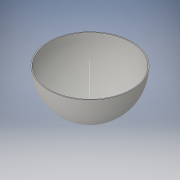
# Autodesk Inventor part: roundSaladBowl
Saved by Autodesk Inventor 2016 SP1 (Build 200210100, 210)
## iProperties
Created: 2016-01-19
Part Number: roundSaladBowl
Material: Generic
Document SubType Name: Modeling
Designer: steele
Density: 1 g/cm^3
Appearance: Default
Author: steele
Autodesk Inventor part; units mm, degrees
ref_plane "YZ Plane" through (0, 0, 0) normal (1, 0, 0) x (0, 1, 0)
ref_plane "XZ Plane" through (0, 0, 0) normal (0, 1, 0) x (-1, 0, 0)
ref_plane "XY Plane" through (0, 0, 0) normal (0, 0, 1) x (1, 0, 0)
sketch "Sketch2" plane through (0, 0, 0) normal (0, 0, 1) x (1, 0, 0)
  arc A0 (0, -127) -> (127, 0) centre (0, 0) ccw
  arc A1 (0, -124.46) -> (124.46, 0) centre (0, 0) ccw
  line L0 (124.46, 0) -> (127, 0)
  line L1 (0, -124.46) -> (0, -127)
  line L2 (0, -183.9631) -> (0, 30.6605) projected
  dimension "d1" = 254
  dimension "d2" = 248.92
  constraints: 4 end point, 4 point on circle, 2 centre point, 2 coincident, 1 horizontal
  measures "d1" diameter of A0
  measures "d2" diameter of A1
revolve "Revolution1" add sketch "Sketch2" angle 360 about axis through (0, -10, 0) along (0, 1, 0)
body "Solid1"
